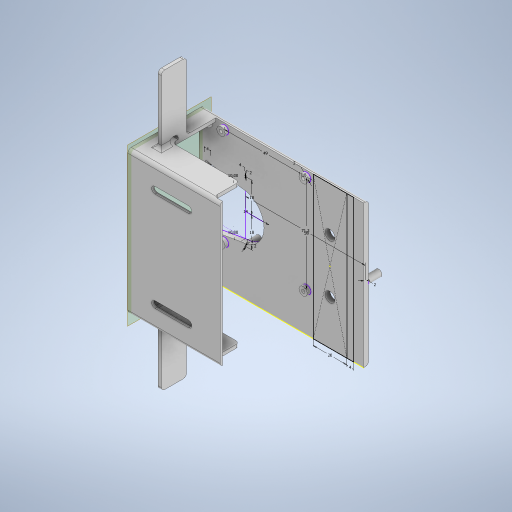
# Autodesk Inventor part: RP4_LidarHolderv4
Saved by Autodesk Inventor 2024 (Build 280153000, 153)
## iProperties
Created: 2025-05-21
Part Number: RP4_LidarHolderv4
Material: Ogólny
Document SubType Name: Modeling
Designer: Victoria
Density: 1 g/cm^3
Appearance: Domyślna
Author: Victoria
Autodesk Inventor part; units mm, degrees
ref_plane "YZ Plane" through (0, 0, 0) normal (1, 0, 0) x (0, 1, 0)
ref_plane "XZ Plane" through (0, 0, 0) normal (0, 1, 0) x (-1, 0, 0)
ref_plane "XY Plane" through (0, 0, 0) normal (0, 0, 1) x (1, 0, 0)
sketch "Szkic1" plane through (0, 0, 0) normal (0, 0, 1) x (1, 0, 0)
  circle A0 centre (0, 16) radius 3
  circle A1 centre (0, -16) radius 3
  line L0 (0, 0) -> (20, 0)
  line L1 (20, 0) -> (20, -42.5)
  line L2 (20, 0) -> (20, 42.5)
  line L3 (20, 0) -> (62.5, 0) construction
  line L4 (20, 42.5) -> (-78, 42.5)
  line L5 (-78, 42.5) -> (-78, -42.5)
  line L6 (-78, -42.5) -> (20, -42.5)
  dimension "d0" = 6
  dimension "d1" = 6
  dimension "d5" = 20
  dimension "d6" = 42.5
  dimension "d7" = 42.5
  dimension "d8" = 90
  dimension "d9" = 98
  dimension "d10" = 85
  dimension "d11" = 90
  constraints: 14 end point, 4 perpendicular, 2 centre point, 2 horizontal, 1 vertical
  measures "d0" diameter of A0
  measures "d1" diameter of A1
  measures "d5" distance of L0.start L0.end
  measures "d6" distance of L0.end L1.end
  measures "d7" distance of L0.end L2.end
  measures "d8" angle of L3 L2
  measures "d9" distance of L2.end L4.end
  measures "d10" distance of L4.end L5.end
  measures "d11" angle of L5 L4
extrude "Wyciągnięcie proste1" add sketch "Szkic1" along normal blind 3
sketch "Szkic2" plane through (0, 0, 3) normal (0, 0, 1) x (1, 0, 0)
  line L0 (-78, -42.5) -> (20, -42.5) projected
  line L1 (-10, 42.5) -> (10, 42.5)
  line L2 (10, 42.5) -> (10, -42.5)
  line L3 (10, -42.5) -> (-10, -42.5)
  line L4 (-10, -42.5) -> (-10, 42.5)
  line L5 (-10, 42.5) -> (10, -42.5) construction
  line L6 (10, 42.5) -> (-10, -42.5) construction
  circle A0 centre (-14, 39) radius 1
  circle A1 centre (-14, 39) radius 2.5
  circle A2 centre (-63, 39) radius 2.5
  circle A3 centre (-63, 39) radius 1
  circle A4 centre (-14, -19) radius 2.5
  circle A5 centre (-14, -19) radius 1
  circle A6 centre (-63, -19) radius 2.5
  circle A7 centre (-63, -19) radius 1
  line L7 (10, 42.5) -> (14, 42.5)
  line L8 (14, 42.5) -> (14, -42.5)
  line L9 (14, -42.5) -> (10, -42.5)
  line L10 (10, -42.5) -> (10, 42.5)
  point P0 (0, 0)
  dimension "d14" = 20
  dimension "d15" = 2
  dimension "d16" = 1.5
  dimension "d19" = 49
  dimension "d22" = 58
  dimension "d25" = 4
  constraints: 20 end point, 8 centre point, 4 parallel, 3 horizontal, 2 midpoint, 2 perpendicular, 2 point on line, 1 vertical, 9 other
  measures "d14" distance of L2.end L3.end
  measures "d15" diameter of A0
  measures "d16" radial gap between concentric circles of A0 A1
  measures "d19" distance of A0.centre A2.centre
  measures "d22" distance of A0.centre A4.centre
  measures "d25" distance of L8.end L9.end
extrude "Wyciągnięcie proste2" add sketch "Szkic2" along normal blind 2 contours A1 | A2 | A4 | A6
extrude "Wyciągnięcie proste3" cut sketch "Szkic2" against normal blind 3 contours A0 | A3 | A5 | A7
sketch "Szkic4" plane through (0, 0, 3) normal (0, 0, 1) x (1, 0, 0)
  line L0 (-78, 42.5) -> (-78, -42.5) projected
  line L1 (-78, -42.5) -> (-68, -42.5)
  line L2 (-68, -42.5) -> (-68, -40.5)
  line L3 (-68, -40.5) -> (-78, -40.5)
  line L4 (-78, -40.5) -> (-78, -42.5)
  line L5 (-78, 42.5) -> (-68, 42.5)
  line L6 (-68, 42.5) -> (-68, 40.5)
  line L7 (-68, 40.5) -> (-78, 40.5)
  line L8 (-78, 40.5) -> (-78, 42.5)
  point P0 (0, 0)
  dimension "d31" = 10
  dimension "d32" = 2
  dimension "d33" = 10
  dimension "d34" = 2
  constraints: 16 end point, 4 parallel, 2 horizontal, 2 perpendicular
  measures "d31" distance of L3.end L2.end
  measures "d32" distance of L2.end L1.end
  measures "d33" distance of L6.end L7.end
  measures "d34" distance of L5.end L6.end
extrude "Wyciągnięcie proste4" add sketch "Szkic4" along normal blind 42.5
sketch "Szkic5" plane through (0, 0, 45.5) normal (0, 0, 1) x (1, 0, 0)
  line L0 (-78, -42.5) -> (20, -42.5) projected
  line L1 (20, 42.5) -> (-78, 42.5) projected
  line L2 (-78, -42.5) -> (-23, -42.5)
  line L3 (-23, -42.5) -> (-23, 42.5)
  line L4 (-23, 42.5) -> (-78, 42.5)
  line L5 (-78, 42.5) -> (-78, -42.5)
  line L6 (-51.815, 0) -> (-51.815, 29.5)
  line L7 (-51.815, 29.5) -> (-51.815, -29.5)
  line L8 (-41.815, -29.5) -> (-61.815, -29.5) construction
  line L9 (-41.815, -27.5) -> (-61.815, -27.5)
  line L10 (-61.815, -31.5) -> (-41.815, -31.5)
  arc A0 (-41.815, -31.5) -> (-41.815, -27.5) centre (-41.815, -29.5) ccw
  arc A1 (-61.815, -27.5) -> (-61.815, -31.5) centre (-61.815, -29.5) ccw
  line L11 (-41.815, 29.5) -> (-61.815, 29.5) construction
  line L12 (-41.815, 31.5) -> (-61.815, 31.5)
  line L13 (-61.815, 27.5) -> (-41.815, 27.5)
  arc A2 (-41.815, 27.5) -> (-41.815, 31.5) centre (-41.815, 29.5) ccw
  arc A3 (-61.815, 31.5) -> (-61.815, 27.5) centre (-61.815, 29.5) ccw
  circle A4 centre (0, 16) radius 3 projected
  circle A5 centre (0, -16) radius 3 projected
  line L14 (0, 0) -> (-22.7, 0)
  dimension "d37" = 55
  dimension "d38" = 29.5
  dimension "d39" = 59
  dimension "d40" = 10
  dimension "d41" = 4
  dimension "d42" = 4
  dimension "d60" = 22.7
  constraints: 30 end point, 8 point on circle, 8 tangent, 5 parallel, 4 centre point, 2 horizontal, 2 midpoint, 2 perpendicular, 2 point on line, 1 vertical
  measures "d37" distance of L4.end L3.end
  measures "d38" distance of L6.start L6.end
  measures "d39" distance of L6.end L7.end
  measures "d40" distance of L7.end L8.end
  measures "d41" diameter of A1
  measures "d42" diameter of A3
  measures "d60" distance of L14.start L14.end
extrude "Wyciągnięcie proste5" add sketch "Szkic5" against normal blind 1.5 contours L5 L1 L3 L0
sketch "Szkic6" plane through (0, 0, 0) normal (0, 0, -1) x (-1, 0, 0)
  circle A0 centre (-18, 0) radius 2
  circle A1 centre (-18, 0) radius 1
  line L0 (-18, 0) -> (53.3, 0)
  line L1 (53.3, 0) -> (53.3, 18)
  line L2 (53.3, 0) -> (53.3, -18)
  circle A2 centre (53.3, -18) radius 1
  circle A3 centre (53.3, -18) radius 2
  circle A4 centre (53.3, 18) radius 1
  circle A5 centre (53.3, 18) radius 2
  arc A6 (53.3, 14) -> (53.3, -14) centre (53.3, 0) ccw
  line L3 (53.3, -14) -> (78, -18.3553)
  line L4 (78, 40.5) -> (78, -40.5) projected
  line L5 (53.3, -14) -> (78.381, -14) construction
  line L6 (53.3, 14) -> (78, 18.3553)
  line L7 (53.3, 14) -> (78.381, 14) construction
  line L8 (78, 18.3553) -> (78, -18.3553)
  line L9 (78, -18.3553) -> (74, -18.3553)
  line L10 (74, -18.3553) -> (74, 18.3553)
  line L11 (74, 18.3553) -> (78, 18.3553)
  line L12 (78, 18.3553) -> (78, -18.3553)
  point P0 (0, 0)
  point P1 (74, -17.65)
  point P2 (74, 17.65)
  dimension "d45" = 2
  dimension "d46" = 71.3
  dimension "d47" = 18
  dimension "d48" = 18
  dimension "d49" = 2
  dimension "d50" = 4
  dimension "d51" = 2
  dimension "d52" = 4
  dimension "d53" = 14
  dimension "d54" = 10
  dimension "d55" = 10
  dimension "d86" = 4
  constraints: 24 end point, 7 centre point, 6 coincident, 4 horizontal, 4 point on line, 2 equal length, 2 parallel, 2 point on circle, 2 vertical, 1 collinear, 1 perpendicular
  measures "d45" diameter of A1
  measures "d46" distance of L0.start L0.end
  measures "d47" distance of L0.end L1.end
  measures "d48" distance of L0.end L2.end
  measures "d49" diameter of A2
  measures "d50" diameter of A3
  measures "d51" diameter of A4
  measures "d52" diameter of A5
  measures "d53" radius of A6
  measures "d54" angle of L3 L5
  measures "d55" angle of L7 L6
  measures "d86" distance of L10.end L11.end
extrude "Wyciągnięcie proste6" add sketch "Szkic6" along normal blind 8 contours A0 | A5 | A3
extrude "Wyciągnięcie proste7" cut sketch "Szkic6" against normal blind 3 contours A6 L1 L0 | L0 L2 A6 | L1 L6 L10 L3 L2
sketch "Szkic7" plane through (-68, 40.5, 3) normal (1, 0, 0) x (0, 0, -1)
  line L0 (-41, 2) -> (-41, -83) projected
  line L1 (0, 0) -> (-41, 0) projected
  line L2 (-41, 2) -> (-26, 2)
  line L3 (-26, 2) -> (-26, 0)
  line L4 (-26, 0) -> (-41, 0)
  line L5 (-41, 0) -> (-41, 2)
  line L6 (-41, -81) -> (-41, -83) projected
  line L7 (0, -83) -> (-41, -83) projected
  line L8 (0, -81) -> (0, -83) projected
  line L9 (0, -81) -> (-41, -81) projected
  line L10 (-41, -83) -> (-26, -83)
  line L11 (-26, -83) -> (-26, -81)
  line L12 (-26, -81) -> (-41, -81)
  line L13 (-41, -81) -> (-41, -83)
  point P0 (3, -40.5)
  dimension "d61" = 15
  dimension "d62" = 15
  constraints: 16 end point, 4 parallel, 2 horizontal, 2 perpendicular, 2 point on line
  measures "d61" distance of L3.end L4.end
  measures "d62" distance of L12.end L11.end
extrude "Wyciągnięcie proste8" add sketch "Szkic7" along normal blind 40 contours L2 L3 L1 L0 | L9 L11 L7 L0
fillet "Zaokrąglenie2" radius 2 6 edges at (-28, 41.5, 29) (-28, 41.5, 44) (-68, 41.5, 29) (-28, -41.5, 44) (-68, -41.5, 29) (-28, -41.5, 29)
sketch "Szkic8" plane through (-78, -42.5, 0) normal (0, -1, 0) x (1, 0, 0)
  arc A0 (12, 29) -> (10, 27) centre (12, 27) ccw projected
  line L0 (10, 27) -> (10, 45.5)
  line L1 (55, 45.5) -> (0, 45.5) projected
  line L2 (10, 45.5) -> (10, 35.5)
  line L3 (10, 35.5) -> (8, 35.5)
  line L4 (8, 35.5) -> (8, 20.5)
  line L5 (8, 20.5) -> (10, 20.5)
  line L6 (10, 20.5) -> (10, 35.5)
  point P0 (78, 0)
  point P1 (10, 27)
  dimension "d68" = 10
  dimension "d69" = 2
  dimension "d70" = 15
  constraints: 12 end point, 2 parallel, 2 point on line, 1 horizontal, 1 perpendicular, 1 vertical
  measures "d68" distance of L0.end L2.end
  measures "d69" distance of L5.end L4.end
  measures "d70" distance of L4.end L3.end
extrude "Wyciągnięcie proste9" add sketch "Szkic8" along normal blind 40
sketch "Szkic9" plane through (-78, 42.5, 0) normal (0, 1, 0) x (1, 0, 0)
  line L0 (8, -20.5) -> (8, -35.5) projected
  line L1 (8, -35.5) -> (8, -20.5) projected
  line L2 (10, -3) -> (10, -27) projected
  line L3 (10, -20.5) -> (10, -35.5) projected
  line L4 (10, -35.5) -> (8, -35.5) projected
  line L5 (8, -35.5) -> (8, -20.5) projected
  line L6 (8, -20.5) -> (10, -20.5) projected
  point P0 (78, 0)
extrude "Wyciągnięcie proste10" add sketch "Szkic9" along normal blind 40
fillet "Zaokrąglenie3" radius 2 8 edges at (-69, 42.5, 20.5) (-69, 42.5, 35.5) (-69, 82.5, 35.5) (-69, 82.5, 20.5) (-69, -42.5, 20.5) (-69, -42.5, 35.5) (-69, -82.5, 20.5) (-69, -82.5, 35.5)
sketch "Szkic10" plane through (-70, -42.5, 18.5) normal (-1, 0, 0) x (0, 0, 1)
  line L0 (9, -3) -> (10, -3)
  line L1 (12, -1) -> (12, 0)
  line L2 (12, 0) -> (7, 0)
  line L3 (7, 0) -> (7, -1)
  arc A0 (7, -1) -> (9, -3) centre (9, -1) ccw
  arc A1 (10, -3) -> (12, -1) centre (10, -1) ccw
  point P0 (-18.5, 42.5)
  dimension "d76" = 5
  dimension "d77" = 2
  constraints: 8 end point, 4 point on circle, 4 tangent, 2 centre point, 2 parallel, 1 equal radius, 1 horizontal, 1 perpendicular
  measures "d76" distance of L2.end L1.end
  measures "d77" radius of A0
extrude "Wyciągnięcie proste11" cut sketch "Szkic10" against normal blind 40
sketch "Szkic11" plane through (-70, 42.5, 18.5) normal (-1, 0, 0) x (0, 0, 1)
  line L0 (19, 0) -> (0, 0) projected
  line L1 (7, 0) -> (12, 0)
  line L2 (12, 0) -> (12, 1)
  line L3 (10, 3) -> (9, 3)
  line L4 (7, 1) -> (7, 0)
  arc A0 (9, 3) -> (7, 1) centre (9, 1) ccw
  arc A1 (12, 1) -> (10, 3) centre (10, 1) ccw
  point P0 (-18.5, -42.5)
  point P1 (12, 3)
  point P2 (7, 3)
  point P3 (12, 0)
  dimension "d80" = 5
  dimension "d81" = 3
  dimension "d82" = 2
  constraints: 8 end point, 5 point on line, 4 point on circle, 4 tangent, 2 centre point, 2 parallel, 1 equal radius, 1 horizontal, 1 perpendicular
  measures "d80" distance of point (7, 3) point (12, 3)
  measures "d81" distance of point (12, 3) L1.end
  measures "d82" radius of A0
extrude "Wyciągnięcie proste12" cut sketch "Szkic11" against normal blind 40
fillet "Zaokrąglenie4" radius 2 6 edges at (-70, 42.5, 34) (-70, 42.5, 22) (-68, 42.5, 34) (-68, -42.5, 34) (-70, -42.5, 34) (-70, -42.5, 22)
sketch "Szkic12" plane through (-78, -42.5, 0) normal (-1, 0, 0) x (0, 0, 1)
  point P0 (0, 42.5)
  point P1 (44, 2)
fillet "Zaokrąglenie5" radius 2 4 edges at (-29, -42.5, 0) (-50.5, -42.5, 45.5) (-50.5, 42.5, 45.5) (-29, 42.5, 0)
ref_plane "Płaszczyzna konstrukcyjna1" through (-76, -40.5, 0) normal (-1, 0, 0) x (0, 0, 1)
sketch "Szkic13" plane through (-76, -40.5, 0) normal (-1, 0, 0) x (0, 0, 1)
  line L0 (3, 81) -> (3, 0) projected
  line L1 (3, 0) -> (44, 0) projected
  circle A0 centre (4, 1) radius 1
  circle A1 centre (4, 1) radius 2.5
  circle A2 centre (4, 80) radius 1
  line L2 (3, 81) -> (44, 81) projected
  circle A3 centre (4, 80) radius 2.5
  point P0 (0, 40.5)
  point P1 (6.2913, 81)
  point P2 (4, 81)
  point P3 (3, 80)
  point P4 (3, 77.7087)
  point P5 (4, 0)
  point P6 (3, 1)
  point P7 (3, 3.2913)
  point P8 (6.2913, 0)
  dimension "d91" = 1.5
  dimension "d92" = 1.5
  constraints: 4 centre point, 2 tangent
  measures "d91" radial gap between concentric circles of A0 A1
  measures "d92" radial gap between concentric circles of A2 A3
extrude "Wyciągnięcie proste13" add sketch "Szkic13" against normal blind 6 contours L2 A2 L0 | A2 L2 A3 L0 | A1 L1 A0 L0 | A0 L1 L0
sketch "Szkic14" plane through (-76, -40.5, 0) normal (-1, 0, 0) x (0, 0, 1)
  line L0 (44, 0) -> (44, 81) projected
  line L1 (44, 0) -> (29, 0)
  line L2 (29, 0) -> (29, 2)
  line L3 (29, 2) -> (44, 2)
  line L4 (44, 2) -> (44, 0)
  line L5 (3, 81) -> (44, 81) projected
  line L6 (44, 81) -> (29, 81)
  line L7 (29, 81) -> (29, 79)
  line L8 (29, 79) -> (44, 79)
  line L9 (44, 79) -> (44, 81)
  point P0 (0, 40.5)
  point P1 (44, 2)
  dimension "d95" = 15
  dimension "d96" = 2
  dimension "d97" = 15
  dimension "d98" = 2
  constraints: 16 end point, 4 parallel, 2 horizontal, 2 perpendicular
  measures "d95" distance of L2.end L3.end
  measures "d96" distance of L1.end L2.end
  measures "d97" distance of L8.end L7.end
  measures "d98" distance of L7.end L6.end
extrude "Wyciągnięcie proste14" add sketch "Szkic14" against normal blind 6
fillet "Zaokrąglenie6" radius 2 4 edges at (-73, -40.5, 29) (-73, -38.5, 29) (-73, 40.5, 29) (-73, 38.5, 29)
